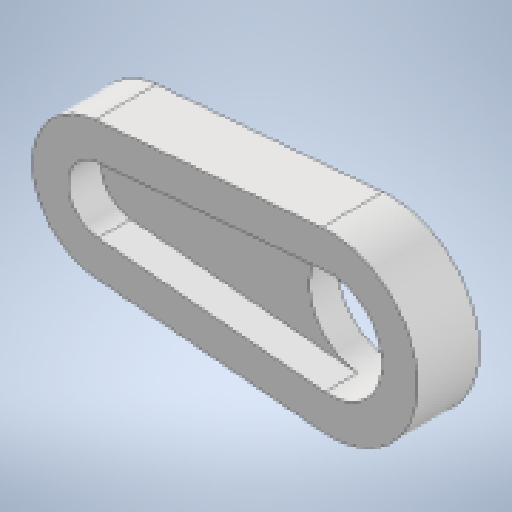
# Autodesk Inventor part: Part37
Saved by Autodesk Inventor 2025.1 (Build 291241000, 241)
## iProperties
Created: 2025-06-18
Part Number: Part37
Material: Generic
Document SubType Name: Modeling
Designer: User
Density: 1 g/cm^3
Appearance: Default
Author: User
## iProperties of the stored document GripperLeft_3DPrint.ipt
Created: 2025-06-19
Part Number: GripperLeft_3DPrint
Material: Generic
Document SubType Name: Modeling
Designer: User
Density: 1 g/cm^3
Appearance: Default
Author: User
Autodesk Inventor part; units mm, degrees
ref_plane "YZ Plane" through (0, 0, 0) normal (1, 0, 0) x (0, 1, 0)
ref_plane "XZ Plane" through (0, 0, 0) normal (0, 1, 0) x (-1, 0, 0)
ref_plane "XY Plane" through (0, 0, 0) normal (0, 0, 1) x (1, 0, 0)
sketch "Sketch1" plane through (0, 0, 0) normal (0, 0, 1) x (1, 0, 0)
  line L0 (6.7664, -3.387) -> (-9.1111, -1.9923) projected
  line L1 (6.7664, 3.387) -> (-9.1111, 1.9923) projected
  arc A0 (-9.1111, 1.9923) -> (-9.1111, -1.9923) centre (-8.9361, 0) ccw projected
  circle A1 centre (-5.2361, 0) radius 0.5 projected
  circle A2 centre (-7.1361, 0) radius 0.5 projected
  circle A3 centre (-9.0361, 0) radius 0.5 projected
  circle A4 centre (2.3639, 0) radius 0.5 projected
  circle A5 centre (0.4639, 0) radius 0.5 projected
  circle A6 centre (-1.4361, 0) radius 0.5 projected
  circle A7 centre (-3.3361, 0) radius 0.5 projected
  arc A8 (6.7664, -3.387) -> (6.7664, 3.387) centre (7.0639, 0) ccw
  line L2 (-9.1373, 2.2912) -> (6.7402, 3.6858)
  arc A9 (6.7402, -3.6858) -> (6.7402, 3.6858) centre (7.0639, 0) ccw
  line L3 (6.7402, -3.6858) -> (-9.1373, -2.2912)
  arc A10 (-9.1373, 2.2912) -> (-9.1373, -2.2912) centre (-8.9361, 0) ccw
  line L4 (6.5214, 6.1762) -> (-9.3561, 4.7816)
  arc A11 (-9.3561, 4.7816) -> (-9.3561, -4.7816) centre (-8.9361, 0) ccw
  line L5 (-9.3561, -4.7816) -> (6.5214, -6.1762)
  arc A12 (6.5214, -6.1762) -> (6.5214, 6.1762) centre (7.0639, 0) ccw
  point P0 (0, 0)
  dimension "d0" = 0.3
  dimension "d1" = 2.5
  constraints: 10 end point, 10 point on circle, 5 centre point, 6 other
  measures "d0" distance between parallel lines of L1 L2
  measures "d1" radial gap between concentric circles of A9 A12
ref_plane "Work Plane1" through (3.5948, -3.4691, -4.3) normal (0, 0, -1) x (0, 1, 0)
extrude "Extrusion1" add sketch "Sketch1" against normal up to surface (4.3 mm away) contours A12 L5 A11 L4
sketch "Sketch2" plane through (7.0639, 0, -4.3) normal (0, 0, -1) x (-1, 0, 0)
  line L0 (0.3238, -3.6858) -> (16.2013, -2.2912) projected
  arc A0 (16.2013, -2.2912) -> (16.2012, 2.2912) centre (16, 0) ccw projected
  line L1 (16.2012, 2.2912) -> (0.3237, 3.6858) projected
  arc A1 (0.2975, -3.387) -> (0.2975, 3.387) centre (0, 0) ccw projected
  circle A2 centre (0, 0) radius 3.7
  point P0 (7.0639, 0)
  point P1 (0.3237, 3.6858)
  constraints: 1 coincident, 3 other
extrude "Extrusion2" add sketch "Sketch2" against normal blind 2 contours A2 L1 A0 L0
sketch "Sketch6" plane through (0, 0, 0) normal (0, 0, 1) x (1, 0, 0)
  circle A0 centre (-13.2269, 5.8971) radius 0.5
  circle A1 centre (-13.2269, 5.8971) radius 1.5
  arc A2 (-9.3561, 4.7816) -> (-9.3561, -4.7816) centre (-8.9361, 0) ccw projected
  line L0 (6.5214, 6.1762) -> (-9.3561, 4.7816) projected
  circle A3 centre (-13.2269, 5.8971) radius 3
  line L1 (-16.0133, 4.7853) -> (-13.3943, -1.7788)
  arc A4 (-10.6035, 7.3522) -> (-6.2746, 5.0523) centre (-6.6683, 9.535) ccw
  point P0 (0, 0)
  dimension "d10" = 3
  dimension "d11" = 6
  dimension "d12" = 9
  constraints: 5 point on circle, 4 centre point, 4 tangent, 2 coincident, 2 end point, 1 point on line, 2 other
  measures "d10" diameter of A1
  measures "d11" diameter of A3
  measures "d12" diameter of A4
extrude "Extrusion5" add sketch "Sketch6" against normal up to surface (4.3 mm away) contours A2 A3 A4 L0 | A2 A3 | A2 L1 A3 picked at (-12.6304, 3.6481)
body "Solid1"
